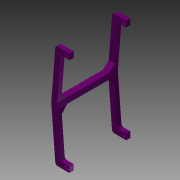
# Autodesk Inventor part: spac
Saved by Autodesk Inventor 2015 (Build 190159000, 159)
## iProperties
Created: 2015-01-15
Part Number: spac
Material: Generic
Document SubType Name: Modeling
Designer: Rafi Kurnia Putra
Density: 1 g/cm^3
Appearance: Smooth - Purple
Author: Rafi Kurnia Putra
Autodesk Inventor part; units mm, degrees
ref_plane "XZ Plane" through (0, 0, 0) normal (0, 1, 0) x (-1, 0, 0)
sketch "Sketch1" plane through (0, 0, 0) normal (0, 1, 0) x (-1, 0, 0)
  circle A0 centre (22.875, -42.175) radius 1.75
  line L0 (20.375, -39.675) -> (20.375, -44.675)
  line L1 (20.375, -44.675) -> (25.375, -44.675)
  line L2 (25.375, -44.675) -> (22.875, -44.675)
  line L3 (30.886, 0) -> (30.886, -2.5058)
  line L4 (35.886, -2.5058) -> (35.886, 0)
  line L5 (35.886, -0.0058) -> (35.886, -2.5058)
  line L6 (34.4637, -0.0058) -> (34.465, 0)
  line L7 (35.886, 0) -> (55.7448, 0) construction
  line L8 (34.4637, 0.0058) -> (34.465, 0)
  line L9 (28.0239, -37.8365) -> (30.886, -2.5058)
  line L10 (35.886, -2.5058) -> (32.6189, -42.8365)
  line L11 (25.375, -44.675) -> (30.6254, -44.675)
  line L12 (20.375, -39.675) -> (26.0305, -39.675)
  line L13 (34.4637, 0.0058) -> (34.465, 0)
  line L14 (34.4637, -0.0058) -> (34.465, 0)
  arc A1 (30.6254, -44.675) -> (32.6189, -42.8365) centre (30.6254, -42.675) ccw
  arc A2 (26.0305, -39.675) -> (28.0239, -37.8365) centre (26.0305, -37.675) ccw
  circle A3 centre (22.875, 42.175) radius 1.75
  line L15 (20.375, 39.675) -> (20.375, 44.675)
  line L16 (20.375, 44.675) -> (25.375, 44.675)
  line L17 (25.375, 44.675) -> (22.875, 44.675)
  line L18 (30.886, 0) -> (30.886, 2.5058)
  line L19 (35.886, 2.5058) -> (35.886, 0)
  line L20 (35.886, 0.0058) -> (35.886, 2.5058)
  line L21 (34.4637, 0.0058) -> (34.465, 0)
  line L22 (34.4637, -0.0058) -> (34.465, 0)
  line L23 (28.0239, 37.8365) -> (30.886, 2.5058)
  line L24 (35.886, 2.5058) -> (32.6189, 42.8365)
  line L25 (25.375, 44.675) -> (30.6254, 44.675)
  line L26 (20.375, 39.675) -> (26.0305, 39.675)
  line L27 (34.4637, -0.0058) -> (34.465, 0)
  line L28 (34.4637, 0.0058) -> (34.465, 0)
  arc A4 (32.6189, 42.8365) -> (30.6254, 44.675) centre (30.6254, 42.675) ccw
  arc A5 (28.0239, 37.8365) -> (26.0305, 39.675) centre (26.0305, 37.675) ccw
  point P0 (0, 0)
  point P1 (27.875, -39.675)
  point P2 (30.886, -2.5058)
  point P3 (35.886, -1.2558)
  point P4 (30.886, -1.2529)
  point P5 (27.875, 39.675)
  point P6 (30.886, 2.5058)
  point P7 (35.886, 1.2558)
  point P8 (30.886, 1.2529)
  dimension "d4" = 3.5
  dimension "d8" = 5
  dimension "d9" = 5
  dimension "d62" = 7.5
  dimension "d63" = 2.5
  dimension "d64" = 2
  constraints: 58 end point, 25 symmetric about line, 8 point on circle, 6 centre point, 6 coincident, 6 point on line, 4 tangent, 2 horizontal, 2 midpoint, 2 parallel, 1 equal radius, 8 other
  measures "d4" diameter of A0
  measures "d8" distance of L1.end L0.end
  measures "d9" distance of L0.start L0.end
  measures "d62" distance of L0.start point (27.875, -39.675)
  measures "d63" distance from line of L0 A0.centre
  measures "d64" radius of A1
extrude "Extrusion11" add sketch "Sketch1" along normal blind 3.5
sketch "Sketch5" plane through (0, 3.5, 0) normal (0, 1, 0) x (1, 0, 0)
  line L0 (-35.886, 2.5058) -> (-30.886, 2.5058)
  line L1 (-30.886, 2.5058) -> (-30.886, -2.4942)
  line L2 (-30.886, -2.4942) -> (-35.886, -2.4942)
  line L3 (-35.886, -2.4942) -> (-35.886, 2.5058)
  point P0 (0, 0)
  dimension "d67" = 5
  dimension "d68" = 5
  constraints: 8 end point, 2 parallel, 1 horizontal, 1 perpendicular
  measures "d67" distance of L1.end L2.end
  measures "d68" distance of L0.end L1.end
extrude "Extrusion12" add sketch "Sketch5" along normal blind 22.75
ref_plane "Work Plane10" through (-33.25, 0, 0) normal (1, 0, 0) x (0, 1, 0)
sketch "Sketch6" plane through (-33.25, 0, 0) normal (1, 0, 0) x (0, 1, 0)
  line L0 (3.5, -2.5058) -> (3.5, -7.5058)
  line L1 (3.5, -2.5058) -> (3.5, -37.8365) projected
  line L2 (3.5, -2.5058) -> (8.5, -2.5058) construction
  line L3 (3.5, -7.5058) -> (8.5, -2.5058)
  line L4 (3.5, -2.5058) -> (26.25, -2.5058) projected
  line L5 (8.5, -2.5058) -> (3.5, -2.5058)
  point P0 (0, 0)
  dimension "d72" = 5
  dimension "d73" = 90
  dimension "d74" = 45
  constraints: 8 end point, 2 perpendicular, 1 collinear, 1 horizontal, 1 point on line
  measures "d72" distance of L0.start L0.end
  measures "d73" angle of L0 L2
  measures "d74" angle of L3 L0
extrude "Extrusion13" add sketch "Sketch6" along normal mid plane 7
ref_plane "Work Plane11" through (0, 0, 0) normal (0, 0, 1) x (1, 0, 0)
mirror "Mirror5" about plane through (0, 0, 0) normal (0, 0, 1) of "Extrusion13"
mirror "Mirror6" about plane through (-33.386, 26.25, -0.0058) normal (0, 1, 0) of "Extrusion11", "Extrusion12", "Extrusion13", "Mirror5"
sketch "Sketch7" plane through (-35.886, 0, -2.5058) normal (-1, 0, 0) x (0, 0, 1)
  line L0 (5.0117, 52.5) -> (0, 52.5)
  line L1 (1.2358, 11.968) -> (1.2358, 12.435)
  spline S0 degree 2 poles (1.2358, 12.435) (1.2358, 12.9021) (1.3086, 13.2332) (1.6053, 13.4419) (1.9287, 13.4419) knots 0 0 0 1 2 3 3 3
  spline S1 degree 2 poles (1.9287, 13.4419) (2.2254, 13.4419) (2.4302, 13.2945) (2.4513, 13.0782) knots 0 0 0 1 2 2 2
  spline S2 degree 2 poles (2.4513, 13.0782) (2.4991, 13.2734) (2.6618, 13.4093) (2.7977, 13.4419) (3.1059, 13.4419) knots 0 0 0 1 2 3 3 3
  line L2 (3.1059, 13.4419) -> (3.7758, 13.4419)
  line L3 (3.7758, 13.4419) -> (3.7758, 12.8274)
  line L4 (3.7758, 12.8274) -> (2.9317, 12.8274)
  spline S3 degree 2 poles (2.9317, 12.8274) (2.7288, 12.8274) (2.6312, 12.7643) (2.6312, 12.6284) knots 0 0 0 1 2 2 2
  line L5 (2.6312, 12.6284) -> (3.7758, 12.6284)
  line L6 (3.7758, 12.6284) -> (3.7758, 11.968)
  line L7 (3.7758, 11.968) -> (1.2358, 11.968)
  line L8 (1.6703, 12.6284) -> (2.235, 12.6284)
  spline S4 degree 2 poles (2.235, 12.6284) (2.235, 12.7394) (2.1737, 12.8274) (2.0053, 12.8274) knots 0 0 0 1 2 2 2
  line L9 (2.0053, 12.8274) -> (1.8656, 12.8274)
  spline S5 degree 2 poles (1.8656, 12.8274) (1.745, 12.8274) (1.6703, 12.7413) (1.6703, 12.6284) knots 0 0 0 1 2 2 2
  spline S6 degree 2 poles (2.7231, 18.0395) (3.1059, 18.0395) (3.4236, 18.0031) (3.6878, 17.8136) (3.8294, 17.4902) (3.8294, 17.2758) knots 0 0 0 1 2 3 4 4 4
  spline S7 degree 2 poles (3.8294, 17.2758) (3.8294, 17.071) (3.6954, 16.7475) (3.4294, 16.5503) (3.1155, 16.5121) (2.7231, 16.5121) knots 0 0 0 1 2 3 4 4 4
  line L10 (2.7231, 16.5121) -> (2.2886, 16.5121)
  spline S8 degree 2 poles (2.2886, 16.5121) (1.9058, 16.5121) (1.588, 16.5484) (1.3239, 16.7379) (1.1822, 17.0614) (1.1822, 17.2758) knots 0 0 0 1 2 3 4 4 4
  spline S9 degree 2 poles (1.1822, 17.2758) (1.1822, 17.4806) (1.3162, 17.8041) (1.5823, 18.0012) (1.8962, 18.0395) (2.2886, 18.0395) knots 0 0 0 1 2 3 4 4 4
  line L11 (2.2886, 18.0395) -> (2.7231, 18.0395)
  spline S10 degree 2 poles (1.8885, 17.3791) (1.7124, 17.3791) (1.6129, 17.3409) (1.6129, 17.2796) knots 0 0 0 1 2 2 2
  spline S11 degree 2 poles (1.6129, 17.2796) (1.6129, 17.2279) (1.6933, 17.1724) (1.8885, 17.1724) knots 0 0 0 1 2 2 2
  line L12 (1.8885, 17.1724) -> (3.0734, 17.1724)
  spline S12 degree 2 poles (3.0734, 17.1724) (3.2954, 17.1724) (3.3988, 17.2088) (3.3988, 17.2739) knots 0 0 0 1 2 2 2
  spline S13 degree 2 poles (3.3988, 17.2739) (3.3988, 17.3409) (3.2801, 17.3791) (3.0561, 17.3791) knots 0 0 0 1 2 2 2
  line L13 (3.0561, 17.3791) -> (1.8885, 17.3791)
  line L14 (1.2358, 21.1193) -> (1.2358, 21.7777)
  spline S14 degree 2 poles (1.2358, 21.7777) (1.2358, 22.0916) (1.3335, 22.4132) (1.6301, 22.6104) (1.9594, 22.6104) knots 0 0 0 1 2 3 3 3
  spline S15 degree 2 poles (1.9594, 22.6104) (2.1814, 22.6104) (2.3575, 22.4706) (2.4034, 22.2639) knots 0 0 0 1 2 2 2
  spline S16 degree 2 poles (2.4034, 22.2639) (2.457, 22.4936) (2.6963, 22.6563) (2.9451, 22.6563) knots 0 0 0 1 2 2 2
  line L15 (2.9451, 22.6563) -> (3.1786, 22.6563)
  spline S17 degree 2 poles (3.1786, 22.6563) (3.437, 22.6563) (3.684, 22.5395) (3.7758, 22.2811) (3.7758, 21.883) knots 0 0 0 1 2 3 3 3
  line L16 (3.7758, 21.883) -> (3.7758, 21.1193)
  line L17 (3.7758, 21.1193) -> (1.2358, 21.1193)
  line L18 (2.6312, 21.7796) -> (3.3413, 21.7796)
  spline S18 degree 2 poles (3.3413, 21.7796) (3.3375, 21.9194) (3.259, 21.9959) (3.104, 21.9959) knots 0 0 0 1 2 2 2
  line L19 (3.104, 21.9959) -> (2.8686, 21.9959)
  spline S19 degree 2 poles (2.8686, 21.9959) (2.7039, 21.9959) (2.635, 21.927) (2.6312, 21.7796) knots 0 0 0 1 2 2 2
  line L20 (1.6703, 21.7796) -> (2.235, 21.7796)
  spline S20 degree 2 poles (2.235, 21.7796) (2.2331, 21.8217) (2.2331, 21.8447) knots 0 0 0 1 1 1
  spline S21 degree 2 poles (2.2331, 21.8447) (2.2331, 21.9423) (2.1374, 21.9959) (1.9115, 21.9959) knots 0 0 0 1 2 2 2
  spline S22 degree 2 poles (1.9115, 21.9959) (1.7928, 21.9959) (1.6971, 21.9519) (1.6722, 21.8811) (1.6703, 21.7796) knots 0 0 0 1 2 3 3 3
  line L21 (1.2358, 27.2271) -> (2.9336, 27.2271)
  spline S23 degree 2 poles (2.9336, 27.2271) (3.2227, 27.2271) (3.4562, 27.1889) (3.7031, 27.0051) (3.8294, 26.7027) (3.8294, 26.496) knots 0 0 0 1 2 3 4 4 4
  spline S24 degree 2 poles (3.8294, 26.496) (3.8294, 26.2682) (3.6782, 25.9217) (3.437, 25.7476) (3.1691, 25.7169) (2.7384, 25.7169) knots 0 0 0 1 2 3 4 4 4
  line L22 (2.7384, 25.7169) -> (1.2358, 25.7169)
  line L23 (1.2358, 25.7169) -> (1.2358, 26.3773)
  line L24 (1.2358, 26.3773) -> (3.1404, 26.3773)
  spline S25 degree 2 poles (3.1404, 26.3773) (3.3069, 26.3773) (3.3988, 26.4137) (3.3988, 26.4672) knots 0 0 0 1 2 2 2
  spline S26 degree 2 poles (3.3988, 26.4672) (3.3988, 26.5304) (3.2973, 26.5668) (3.1078, 26.5668) knots 0 0 0 1 2 2 2
  line L25 (3.1078, 26.5668) -> (1.2358, 26.5668)
  line L26 (1.2358, 26.5668) -> (1.2358, 27.2271)
  line L27 (2.0034, 31.7157) -> (2.0034, 31.1013)
  line L28 (2.0034, 31.1013) -> (1.8158, 31.1013)
  spline S27 degree 2 poles (1.8158, 31.1013) (1.6856, 31.1013) (1.6129, 31.0553) (1.6129, 30.9998) knots 0 0 0 1 2 2 2
  spline S28 degree 2 poles (1.6129, 30.9998) (1.6129, 30.9405) (1.7105, 30.8792) (1.8081, 30.8792) knots 0 0 0 1 2 2 2
  spline S29 degree 2 poles (1.8081, 30.8792) (1.9345, 30.8792) (1.9996, 30.9137) knots 0 0 0 1 1 1
  spline S30 degree 2 poles (1.9996, 30.9137) (2.0646, 30.9481) (2.1546, 31.1013) knots 0 0 0 1 1 1
  spline S31 degree 2 poles (2.1546, 31.1013) (2.4168, 31.5415) (2.5853, 31.6564) knots 0 0 0 1 1 1
  spline S32 degree 2 poles (2.5853, 31.6564) (2.7537, 31.7712) (3.127, 31.7712) knots 0 0 0 1 1 1
  spline S33 degree 2 poles (3.127, 31.7712) (3.3988, 31.7712) (3.6552, 31.6449) (3.8294, 31.2793) (3.8294, 31.0381) knots 0 0 0 1 2 3 3 3
  spline S34 degree 2 poles (3.8294, 31.0381) (3.8294, 30.774) (3.6284, 30.3988) (3.3184, 30.282) (3.0332, 30.282) knots 0 0 0 1 2 3 3 3
  line L29 (3.0332, 30.282) -> (2.8666, 30.282)
  line L30 (2.8666, 30.282) -> (2.8666, 30.8965)
  line L31 (2.8666, 30.8965) -> (3.1748, 30.8965)
  spline S35 degree 2 poles (3.1748, 30.8965) (3.3164, 30.8965) (3.3988, 30.9481) (3.3988, 31.0132) knots 0 0 0 1 2 2 2
  spline S36 degree 2 poles (3.3988, 31.0132) (3.3988, 31.0802) (3.2954, 31.1434) (3.1939, 31.1434) knots 0 0 0 1 2 2 2
  spline S37 degree 2 poles (3.1939, 31.1434) (2.97, 31.1434) (2.9011, 31.0821) knots 0 0 0 1 1 1
  spline S38 degree 2 poles (2.9011, 31.0821) (2.8322, 31.019) (2.6695, 30.772) knots 0 0 0 1 1 1
  spline S39 degree 2 poles (2.6695, 30.772) (2.5068, 30.527) (2.3594, 30.3663) (2.0991, 30.261) (1.8962, 30.261) knots 0 0 0 1 2 3 3 3
  spline S40 degree 2 poles (1.8962, 30.261) (1.6033, 30.261) (1.3335, 30.4103) (1.1822, 30.7433) (1.1822, 30.9788) knots 0 0 0 1 2 3 3 3
  spline S41 degree 2 poles (1.1822, 30.9788) (1.1822, 31.2353) (1.3488, 31.5989) (1.6014, 31.7157) (1.9038, 31.7157) knots 0 0 0 1 2 3 3 3
  line L32 (1.9038, 31.7157) -> (2.0034, 31.7157)
  line L33 (1.2358, 36.1411) -> (1.745, 36.1411)
  line L34 (1.745, 36.1411) -> (1.745, 35.7487)
  line L35 (1.745, 35.7487) -> (3.7758, 35.7487)
  line L36 (3.7758, 35.7487) -> (3.7758, 35.0883)
  line L37 (3.7758, 35.0883) -> (1.745, 35.0883)
  line L38 (1.745, 35.0883) -> (1.745, 34.6978)
  line L39 (1.745, 34.6978) -> (1.2358, 34.6978)
  line L40 (1.2358, 34.6978) -> (1.2358, 36.1411)
  line L41 (1.2358, 40.2659) -> (3.7758, 40.6449)
  line L42 (3.7758, 40.6449) -> (3.7758, 39.9673)
  line L43 (3.7758, 39.9673) -> (3.3184, 39.9329)
  line L44 (3.3184, 39.9329) -> (3.3184, 39.6975)
  line L45 (3.3184, 39.6975) -> (3.7758, 39.6592)
  line L46 (3.7758, 39.6592) -> (3.7758, 38.9739)
  line L47 (3.7758, 38.9739) -> (1.2358, 39.3089)
  line L48 (1.2358, 39.3089) -> (1.2358, 40.2659)
  spline S42 degree 2 poles (2.8686, 39.9157) (2.4379, 39.8678) (1.8024, 39.8161) knots 0 0 0 1 1 1
  spline S43 degree 2 poles (1.8024, 39.8161) (2.5317, 39.7166) (2.8686, 39.6898) knots 0 0 0 1 1 1
  line L49 (2.8686, 39.6898) -> (2.8686, 39.9157)
  point P0 (2.5058, 0)
  point P1 (2.5058, 26.25)
  point P2 (5, 49)
  point P3 (0.5, 49)
  point P4 (0.5, 0)
  point P5 (0, 44)
  point P6 (0, 8.5)
  point P7 (5.0117, 8.5)
  point P8 (2.5058, 26.25)
  point P9 (2.5058, 26.25)
  constraints: 2 end point, 1 coincident, 2 other
sketch "Sketch8" plane through (-30.886, 3.5, -2.5058) normal (0, -1, 0) x (1, 0, 0)
  line L0 (1.136, 0) -> (1.136, -5)
  line L1 (1.136, -5) -> (0.405, -5)
  line L2 (2.8621, -35.3307) -> (0, 0) projected
  line L3 (0, 0) -> (1.136, 0)
  line L4 (0, 0) -> (1.136, 0) projected
  point P0 (30.886, 2.5058)
  constraints: 6 end point, 1 collinear, 1 perpendicular, 1 point on line, 1 vertical
extrude "Extrusion15" cut sketch "Sketch8" against normal through all
sketch "Sketch9" plane through (-36.75, 3.5, -7.5058) normal (0, -1, 0) x (1, 0, 0)
  line L0 (0, 5) -> (0.364, 5)
  arc A0 (0.364, 5) -> (0.8367, 5.337) centre (0.364, 5.5) ccw
  arc A1 (0.8367, 5.337) -> (0.864, 5.5) centre (0.364, 5.5) ccw projected
  line L1 (0.864, 5.5) -> (1.269, 0)
  line L2 (1.269, 0) -> (0, 0)
  line L3 (0, 0) -> (1.269, 0) projected
  line L4 (0, 0) -> (0, 5)
  point P0 (36.75, 7.5058)
  constraints: 8 end point, 3 point on circle, 1 centre point, 1 collinear, 1 horizontal, 1 perpendicular
extrude "Extrusion16" cut sketch "Sketch9" against normal through all
sketch "Sketch10" plane through (-30.886, 3.5, 2.5058) normal (0, -1, 0) x (1, 0, 0)
  line L0 (1.136, 5) -> (1.136, 0)
  line L1 (1.136, 0) -> (1.136, 5) projected
  line L2 (1.136, 0) -> (0, -0.0117)
  line L3 (0, -0.0117) -> (0.405, 5)
  line L4 (0, 0) -> (2.8621, 35.3307) projected
  line L5 (1.136, 5) -> (0.405, 5)
  line L6 (0.405, 5) -> (0, 0)
  line L7 (1.136, 0) -> (1.136, 5)
  point P0 (30.886, -2.5058)
  constraints: 12 end point, 2 collinear, 1 horizontal, 1 point on line
extrude "Extrusion17" cut sketch "Sketch10" against normal through all
sketch "Sketch11" plane through (-36.75, 3.5, 7.5058) normal (0, -1, 0) x (1, 0, 0)
  line L0 (1.269, 0) -> (0.864, -5)
  line L1 (0.864, -5) -> (1.269, 0) projected
  line L2 (0.864, -5) -> (0, -5)
  line L3 (0.864, -5) -> (0, -5) projected
  line L4 (0, -5) -> (0, 0)
  line L5 (0, 0) -> (1.269, 0)
  line L6 (0, 0) -> (1.269, 0) projected
  point P0 (36.75, -7.5058)
  constraints: 8 end point, 3 collinear, 1 perpendicular
extrude "Extrusion18" cut sketch "Sketch11" against normal through all
extrude "Extrusion19" add sketch "Sketch7" along normal blind 1.5
body "Solid4"
